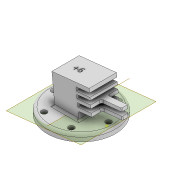
# Autodesk Inventor part: Plate_6
Saved by Autodesk Inventor 2022 (Build 260153000, 153)
## iProperties
Created: 2022-12-25
Part Number: Plate_6
Material: Generic
Document SubType Name: Modeling
Designer: dell
Density: 1 g/cm^3
Appearance: Default
Author: dell
Autodesk Inventor part; units mm, degrees
ref_plane "YZ Plane" through (0, 0, 0) normal (1, 0, 0) x (0, 1, 0)
ref_plane "XZ Plane" through (0, 0, 0) normal (0, 1, 0) x (-1, 0, 0)
ref_plane "XY Plane" through (0, 0, 0) normal (0, 0, 1) x (1, 0, 0)
sketch "Sketch1" plane through (0, 0, 0) normal (0, 1, 0) x (-1, 0, 0)
  circle A0 centre (0, 0) radius 50
  dimension "d0" = 100
  constraints: 1 centre point, 1 coincident
  measures "d0" diameter of A0
extrude "Extrusion1" add sketch "Sketch1" along normal blind 10
sketch "Sketch2" plane through (0, 10, 0) normal (0, 1, 0) x (1, 0, 0)
  circle A0 centre (-40, 0) radius 4.1
  point P0 (0, 0)
  dimension "d3" = 8.2
  dimension "d4" = 40
  constraints: 1 centre point
  measures "d3" diameter of A0
  measures "d4" distance of point (0, 0) A0.centre
extrude "Extrusion2" cut sketch "Sketch2" against normal blind 100
pattern_circular "Circular Pattern1" count 6 over 360 about axis through (0, 0, 0) along (0, 1, 0) of "Extrusion2"
ref_plane "Work Plane1" through (0, 10, -10) normal (0.1045285, -0.9945219, 0) x (0, 0, 1)
sketch "Sketch3" plane through (0, 10, 0) normal (-0.1045285, 0.9945219, 0) x (0.9945219, 0.1045285, 0)
  line L0 (-18.5453, 20) -> (16.4547, 20)
  line L1 (16.4547, 20) -> (16.4547, -20)
  line L2 (16.4547, -20) -> (-18.5453, -20)
  line L3 (-18.5453, -20) -> (-18.5453, 20)
  line L4 (-18.5453, 20) -> (16.4547, -20) construction
  line L5 (16.4547, 20) -> (-18.5453, -20) construction
  point P0 (-1.0453, 0)
  dimension "d10" = 35
  dimension "d11" = 40
  constraints: 12 end point, 2 midpoint, 2 parallel, 1 horizontal, 1 perpendicular
  measures "d10" distance of L1.end L2.end
  measures "d11" distance of L0.end L1.end
extrude "Extrusion3" add sketch "Sketch3" along normal blind 45
sketch "Sketch5" plane through (16.5454, 10, 20) normal (0.9945219, 0.1045285, 0) x (0, 0, -1)
  line L0 (0, 1.7295) -> (0, 46.7295) projected
  line L1 (40, 3.6786) -> (40, 46.7295) projected
  line L2 (0, 16.7295) -> (40, 16.7295)
  line L3 (40, 16.7295) -> (40, 11.7295)
  line L4 (40, 11.7295) -> (0, 11.7295)
  line L5 (0, 11.7295) -> (0, 16.7295)
  line L6 (0, 3.6786) -> (0, 46.7295) projected
  line L7 (0, 21.7295) -> (40, 21.7295)
  line L8 (40, 21.7295) -> (40, 26.7295)
  line L9 (40, 26.7295) -> (0, 26.7295)
  line L10 (0, 26.7295) -> (0, 21.7295)
  line L11 (40, 3.6786) -> (40, 46.7295) projected
  line L12 (0, 35.9295) -> (40, 35.9295)
  line L13 (40, 35.9295) -> (40, 31.7295)
  line L14 (40, 31.7295) -> (0, 31.7295)
  line L15 (0, 31.7295) -> (0, 35.9295)
  line L16 (0, 40.9295) -> (40, 40.9295)
  line L17 (40, 1.7295) -> (40, 46.7295) projected
  line L18 (0, 46.7295) -> (40, 46.7295) projected
  line L19 (0, 1.7295) -> (0, 46.7295) projected
  line L20 (0, 1.7295) -> (40, 1.7295) projected
  point P0 (20, -8.2158)
  point P1 (0, 0)
  point P2 (0, 11.7295)
  point P3 (0, 40.9295)
  point P4 (0, 31.7295)
  point P5 (0, 35.9295)
  point P6 (0, 26.7295)
  point P7 (0, 21.7295)
  dimension "d16" = 5
  dimension "d19" = 5
  dimension "d20" = 5
  dimension "d21" = 5
  dimension "d22" = 4.2
  dimension "d23" = 5
  dimension "d44" = 15
  constraints: 26 end point, 8 point on line, 6 parallel, 4 perpendicular, 3 horizontal
  measures "d16" distance between parallel lines of L2 L4
  measures "d19" distance between parallel lines of L7 L2
  measures "d20" distance between parallel lines of L7 L9
  measures "d21" distance between parallel lines of L9 L14
  measures "d22" distance between parallel lines of L14 L12
  measures "d23" distance between parallel lines of L12 L16
  measures "d44" distance between parallel lines of L20 L2
extrude "Extrusion4" add sketch "Sketch5" along normal blind 20 contours L0 L2 L1 L4 | L0 L9 L1 L7 | L0 L12 L1 L14 | L0 L18 L1 L16
sketch "Sketch7" plane through (36.4358, 12.0906, 20) normal (0.9945219, 0.1045285, 0) x (0, 0, -1)
  point P0 (20, -8.2158)
sketch "Sketch6" plane through (36.4358, 12.0906, 20) normal (0.9945219, 0.1045285, 0) x (0, 0, -1)
  line L0 (40, 11.7295) -> (40, 16.7295) projected
  line L1 (40, 16.7295) -> (0, 16.7295) projected
  line L2 (0, 16.7295) -> (0, 11.7295) projected
  line L3 (0, 11.7295) -> (40, 11.7295) projected
  line L4 (0, 26.7295) -> (0, 21.7295) projected
  line L5 (0, 21.7295) -> (40, 21.7295) projected
  line L6 (40, 21.7295) -> (40, 26.7295) projected
  line L7 (40, 26.7295) -> (0, 26.7295) projected
  line L8 (40, 26.7295) -> (0, 26.7295) projected
  line L9 (15.5, 26.7295) -> (24.5, 26.7295)
  line L10 (24.5, 26.7295) -> (24.5, 21.7295)
  line L11 (24.5, 21.7295) -> (15.5, 21.7295)
  line L12 (15.5, 21.7295) -> (15.5, 26.7295)
  line L13 (40, 16.7295) -> (0, 16.7295) projected
  line L14 (15.5, 16.7295) -> (24.5, 16.7295)
  line L15 (24.5, 16.7295) -> (24.5, 11.7295)
  line L16 (24.5, 11.7295) -> (15.5, 11.7295)
  line L17 (15.5, 11.7295) -> (15.5, 16.7295)
  line L18 (20, -27.1814) -> (20, 68.9931) projected
  point P0 (20, -8.2158)
  point P1 (15.5, 11.7295)
  point P2 (24.5, 26.7295)
  point P3 (15.5, 26.7295)
  dimension "d24" = 9
  dimension "d25" = 9
  dimension "d26" = 4.5
  dimension "d27" = 4.5
  constraints: 16 end point, 4 parallel, 4 point on line, 2 horizontal, 2 perpendicular
  measures "d24" distance between parallel lines of L10 L12
  measures "d25" distance between parallel lines of L17 L15
  measures "d26" distance between parallel lines of L18 L12
  measures "d27" distance between parallel lines of L18 L17
extrude "Extrusion5" add sketch "Sketch6" along normal blind 30 contours L3 L18 L1 L15 | L3 L17 L1 L18 | L7 L18 L5 L12 | L7 L10 L5 L18
thicken "Thicken1" operation add thickness 0.2 both sides no extend neighbours yes toward (0.1045285, -0.9945219, 0) faces at (21.4268, 27.3347, -1.5)
thicken "Thicken2" operation add thickness 0.2 both sides no extend neighbours yes toward (-0.1045285, 0.9945219, 0) faces at (20.9042, 32.3073, -1.5)
thicken "Thicken3" operation add thickness 0.2 both sides no extend neighbours yes toward (0.1045285, -0.9945219, 0) faces at (20.3815, 37.2799, -1.5)
thicken "Thicken4" operation add thickness 0.2 both sides no extend neighbours yes toward (-0.1045285, 0.9945219, 0) faces at (19.8589, 42.2525, -6.6667)
thicken "Thicken5" operation add thickness 0.2 both sides no extend neighbours yes toward (0.1045285, -0.9945219, 0) faces at (26.05, 47.1263, 6.6667)
thicken "Thicken6" operation add thickness 0.2 both sides no extend neighbours yes toward (-0.1045285, 0.9945219, 0) faces at (25.5274, 52.099, 6.6667)
fillet "Fillet1" radius 3 8 edges at (-18.6474, 10, 0) (-9.3237, 10, -20) (-9.3237, 10, 20) (15.3193, 21.6652, 0) (34.9589, 26.1426, -4.5) (33.9031, 36.1873, -4.5) (33.9031, 36.1873, 4.5) (34.9589, 26.1426, 4.5)
chamfer "Chamfer1" distance 14 angle 45 1 edges at (0, 10, 0)
fillet "Fillet3" radius 10 1 edges at (14, 10, 0)
fillet "Fillet4" radius 4 3 edges at (-35.3553, 10, -35.3553) (-35.3553, 10, 35.3553) (50, 10, 0)
sketch "Sketch8" plane through (-4.7038, 54.7535, 0) normal (-0.1045285, 0.9945219, 0) x (0.9945219, 0.1045285, 0)
  line L0 (-6.9685, 4.6888) -> (10.8183, 4.6888) construction
  line L1 (10.8183, 4.6888) -> (10.8183, -13.2224) construction
  line L2 (10.8183, -13.2224) -> (-6.9685, -13.2224) construction
  line L3 (-6.9685, -13.2224) -> (-6.9685, 4.6888) construction
  line L4 (0.1952, -0.3874) -> (-2.5147, -0.3874)
  line L5 (-2.5147, -0.3874) -> (-2.5147, -3.0973)
  line L6 (-2.5147, -3.0973) -> (-3.4093, -3.0973)
  line L7 (-3.4093, -3.0973) -> (-3.4093, -0.3874)
  line L8 (-3.4093, -0.3874) -> (-6.1192, -0.3874)
  line L9 (-6.1192, -0.3874) -> (-6.1192, 0.4748)
  line L10 (-6.1192, 0.4748) -> (-3.4093, 0.4748)
  line L11 (-3.4093, 0.4748) -> (-3.4093, 3.1847)
  line L12 (-3.4093, 3.1847) -> (-2.5147, 3.1847)
  line L13 (-2.5147, 3.1847) -> (-2.5147, 0.4748)
  line L14 (-2.5147, 0.4748) -> (0.1952, 0.4748)
  line L15 (0.1952, 0.4748) -> (0.1952, -0.3874)
  spline S0 degree 2 poles (6.6782, -0.8672) (6.6782, -1.483) (6.2698, -2.5268) (5.9262, -2.8769) knots 0 0 0 1 2 2 2
  spline S1 degree 2 poles (5.9262, -2.8769) (5.5696, -3.2464) (4.6749, -3.6289) (4.1368, -3.6289) knots 0 0 0 1 2 2 2
  spline S2 degree 2 poles (4.1368, -3.6289) (3.5988, -3.6289) (2.7106, -3.2659) (2.3735, -2.9028) knots 0 0 0 1 2 2 2
  spline S3 degree 2 poles (2.3735, -2.9028) (1.9586, -2.4684) (1.4918, -1.0098) (1.4918, 0.0534) knots 0 0 0 1 2 2 2
  spline S4 degree 2 poles (1.4918, 0.0534) (1.4918, 1.0972) (1.9197, 2.7763) (2.367, 3.3987) knots 0 0 0 1 2 2 2
  spline S5 degree 2 poles (2.367, 3.3987) (2.8014, 4.0081) (4.1757, 4.6888) (5.0769, 4.6888) knots 0 0 0 1 2 2 2
  spline S6 degree 2 poles (5.0769, 4.6888) (5.3427, 4.6888) (5.8095, 4.6369) (5.9845, 4.5786) knots 0 0 0 1 2 2 2
  line L16 (5.9845, 4.5786) -> (5.9845, 3.5478)
  line L17 (5.9845, 3.5478) -> (5.9391, 3.5478)
  spline S7 degree 2 poles (5.9391, 3.5478) (5.79, 3.6256) (5.2454, 3.7617) (4.9343, 3.7617) knots 0 0 0 1 2 2 2
  spline S8 degree 2 poles (4.9343, 3.7617) (3.9359, 3.7617) (2.7106, 2.4132) (2.5939, 1.0907) knots 0 0 0 1 2 2 2
  spline S9 degree 2 poles (2.5939, 1.0907) (2.9764, 1.3565) (3.7803, 1.6482) (4.26, 1.6482) knots 0 0 0 1 2 2 2
  spline S10 degree 2 poles (4.26, 1.6482) (4.7268, 1.6482) (5.427, 1.4602) (5.8095, 1.175) knots 0 0 0 1 2 2 2
  spline S11 degree 2 poles (5.8095, 1.175) (6.2503, 0.8444) (6.6782, -0.18) (6.6782, -0.8672) knots 0 0 0 1 2 2 2
  spline S12 degree 2 poles (5.589, -0.9125) (5.589, -0.4198) (5.3297, 0.2479) (5.0445, 0.4813) knots 0 0 0 1 2 2 2
  spline S13 degree 2 poles (5.0445, 0.4813) (4.8305, 0.6499) (4.2989, 0.7601) (4.0202, 0.7601) knots 0 0 0 1 2 2 2
  spline S14 degree 2 poles (4.0202, 0.7601) (3.6441, 0.7601) (2.9375, 0.5332) (2.5939, 0.3192) knots 0 0 0 1 2 2 2
  spline S15 degree 2 poles (2.5939, 0.3192) (2.5874, 0.2025) (2.5745, -0.0179) (2.5745, -0.1864) knots 0 0 0 1 2 2 2
  spline S16 degree 2 poles (2.5745, -0.1864) (2.5745, -1.0163) (2.8986, -2.0341) (3.145, -2.2999) knots 0 0 0 1 2 2 2
  spline S17 degree 2 poles (3.145, -2.2999) (3.3719, -2.5527) (3.8646, -2.7537) (4.1433, -2.7537) knots 0 0 0 1 2 2 2
  spline S18 degree 2 poles (4.1433, -2.7537) (4.7916, -2.7537) (5.589, -1.8331) (5.589, -0.9125) knots 0 0 0 1 2 2 2
  point P0 (-1.0453, 0)
  constraints: 2 other
extrude "Extrusion6" cut sketch "Sketch8" against normal blind 1
fillet "Fillet5" radius 1 4 edges at (64.7945, 29.2785, 4.5) (63.7388, 39.3232, 4.5) (63.7388, 39.3232, -4.5) (64.7945, 29.2785, -4.5)
equation "\"d26\" = 0.5 * d24"
equation "\"d27\" = 0.5 * d25"
body "Solid1"
